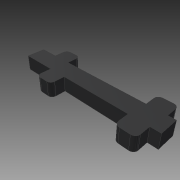
# Autodesk Inventor part: x_motor_smooth_rod_spacer
Saved by Autodesk Inventor 2014 (Build 180170000, 170)
## iProperties
Created: 2013-12-01
Part Number: x_motor_smooth_rod_spacer
Material: Generic
Document SubType Name: Modeling
Designer: buben
Density: 1 g/cm^3
Appearance: Anodized - Dark Gray
Author: buben
Subject: Laser Cutted
Autodesk Inventor part; units mm, degrees
ref_plane "YZ Plane" through (0, 0, 0) normal (1, 0, 0) x (0, 1, 0)
ref_plane "XZ Plane" through (0, 0, 0) normal (0, 1, 0) x (-1, 0, 0)
ref_plane "XY Plane" through (0, 0, 0) normal (0, 0, 1) x (1, 0, 0)
sketch "Sketch1" plane through (0, 0, 0) normal (0, 0, 1) x (1, 0, 0)
  line L0 (0, 0) -> (65, 0)
  line L1 (65, 0) -> (65, 8)
  line L2 (65, 8) -> (0, 8)
  line L3 (0, 8) -> (0, 0)
  dimension "d0" = 8
  dimension "d1" = 65
  constraints: 8 end point, 2 parallel, 1 horizontal, 1 perpendicular
  measures "d0" distance of L2.end L0.start
  measures "d1" distance of L0.start L0.end
extrude "Extrusion1" add sketch "Sketch1" along normal blind 6.5
sketch "Sketch2" plane through (0, 0, 6.5) normal (0, 0, 1) x (1, 0, 0)
  line L0 (0, 0) -> (65, 0) projected
  line L1 (65, 8) -> (0, 8) projected
  line L2 (0, 8) -> (0, 0) projected
  line L3 (15, 0) -> (23, 0)
  line L4 (23, 0) -> (23, -4.5)
  line L5 (21, -6.5) -> (17, -6.5)
  line L6 (15, -4.5) -> (15, 0)
  line L7 (53, 0) -> (61, 0)
  line L8 (61, 0) -> (61, -4.5)
  line L9 (59, -6.5) -> (55, -6.5)
  line L10 (53, -4.5) -> (53, 0)
  line L11 (8, 8) -> (16, 8)
  line L12 (16, 8) -> (16, 12.5)
  line L13 (14, 14.5) -> (10, 14.5)
  line L14 (8, 12.5) -> (8, 8)
  line L15 (54, 8) -> (62, 8)
  line L16 (62, 8) -> (62, 12.5)
  line L17 (60, 14.5) -> (56, 14.5)
  line L18 (54, 12.5) -> (54, 8)
  arc A0 (15, -4.5) -> (17, -6.5) centre (17, -4.5) ccw
  arc A1 (21, -6.5) -> (23, -4.5) centre (21, -4.5) ccw
  arc A2 (10, 14.5) -> (8, 12.5) centre (10, 12.5) ccw
  arc A3 (16, 12.5) -> (14, 14.5) centre (14, 12.5) ccw
  arc A4 (56, 14.5) -> (54, 12.5) centre (56, 12.5) ccw
  arc A5 (62, 12.5) -> (60, 14.5) centre (60, 12.5) ccw
  arc A6 (53, -4.5) -> (55, -6.5) centre (55, -4.5) ccw
  arc A7 (59, -6.5) -> (61, -4.5) centre (59, -4.5) ccw
  dimension "d4" = 2
  dimension "d5" = 8
  dimension "d6" = 6.5
  dimension "d7" = 6.5
  dimension "d8" = 8
  dimension "d9" = 8
  dimension "d10" = 8
  dimension "d11" = 15
  dimension "d12" = 30
  dimension "d13" = 8
  dimension "d14" = 38
  constraints: 32 end point, 16 point on circle, 16 tangent, 8 centre point, 8 parallel, 7 equal radius, 4 horizontal, 4 perpendicular, 4 point on line, 2 collinear
  measures "d4" radius of A0
  measures "d5" distance between parallel lines of L4 L6
  measures "d6" distance between parallel lines of L0 L5
  measures "d7" distance between parallel lines of L1 L13
  measures "d8" distance between parallel lines of L8 L10
  measures "d9" distance between parallel lines of L12 L14
  measures "d10" distance between parallel lines of L16 L18
  measures "d11" distance between parallel lines of L6 L2
  measures "d12" distance between parallel lines of L10 L4
  measures "d13" distance between parallel lines of L2 L14
  measures "d14" distance between parallel lines of L18 L12
extrude "Extrusion2" add sketch "Sketch2" against normal blind 6.5
body "Solid1"
